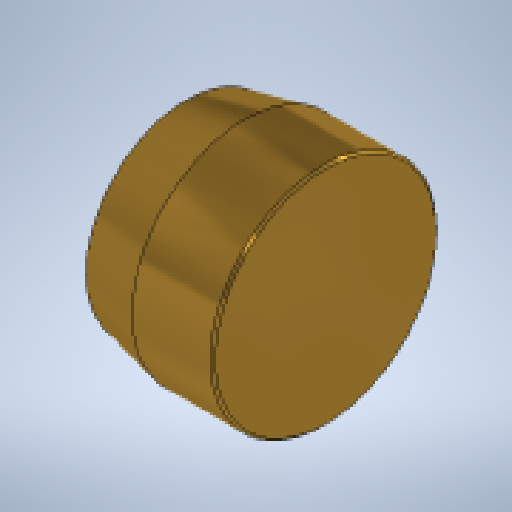
# Autodesk Inventor part: Flywheel
Saved by Autodesk Inventor 2023.2 (Build 272271000, 271)
## iProperties
Created: 2024-01-10
Part Number: Flywheel
Material: Brass, Soft Yellow
Document SubType Name: Modeling
Designer: Nathan Cai
Mass: 167.124 g
Surface Area: 93.7474 cm^2
Volume: 19.7313 cm^3
Density: 8.47 g/cm^3
Appearance: Brass - Satin
Author: Nathan Cai
Autodesk Inventor part; units mm, degrees
ref_plane "YZ Plane" through (0, 0, 0) normal (1, 0, 0) x (0, 1, 0)
ref_plane "XZ Plane" through (0, 0, 0) normal (0, 1, 0) x (-1, 0, 0)
ref_plane "XY Plane" through (0, 0, 0) normal (0, 0, 1) x (1, 0, 0)
sketch "Sketch1" plane through (0, 0, 0) normal (0, 1, 0) x (-1, 0, 0)
  line L0 (0, 0) -> (3.5, 0)
  line L1 (3.5, 0) -> (3.5, -8)
  line L2 (3.5, -8) -> (0, -8)
  line L3 (0, -8) -> (0, 0)
  line L4 (3.5, 0) -> (11.5, 0)
  line L5 (11.5, 0) -> (11.5, -13.9)
  line L6 (11.5, -13.9) -> (3.5, -13.9)
  line L7 (3.5, -13.9) -> (3.5, 0)
  line L8 (0, 0) -> (-13, 0)
  line L9 (-13, 0) -> (-13, -23)
  line L10 (-13, -23) -> (0, -23)
  line L11 (0, -23) -> (0, 0)
  line L12 (-13, -21) -> (0, -18.118)
  line L13 (-13, 0) -> (11.5, 0)
  line L14 (11.5, 0) -> (11.5, -23)
  line L15 (11.5, -23) -> (-13, -23)
  line L16 (-13, -23) -> (-13, 0)
  line L17 (-13, -23) -> (0, -20.118) construction
  line L18 (11.5, -23) -> (15.5, -23)
  line L19 (15.5, -23) -> (15.5, -18.5)
  line L20 (15.5, -18.5) -> (11.5, -18.5)
  line L21 (11.5, -18.5) -> (11.5, -23)
  line L22 (0, -8) -> (-5, -8)
  line L23 (-5, -8) -> (-5, -12)
  line L24 (-5, -12) -> (0, -12)
  line L25 (0, -12) -> (0, -8)
  line L26 (3.5, -8) -> (-2, -8)
  line L27 (-2, -8) -> (-2, -23)
  line L28 (-2, -23) -> (3.5, -23)
  line L29 (3.5, -23) -> (3.5, -8)
  line L30 (-5, -8) -> (-4, -8)
  line L31 (-4, -8) -> (-4, -9.1)
  line L32 (-4, -9.1) -> (-5, -9.1)
  line L33 (-5, -9.1) -> (-5, -8)
  line L34 (15.5, -20.3397) -> (3.5, -23)
  point P0 (3.5, -8)
  point P1 (0, -8)
  point P2 (0, -23)
  point P3 (11.5, -18.5)
  point P4 (0, -12)
  point P5 (0, -8)
  point P6 (0, -23)
  point P7 (3.5, -8)
  point P8 (-2, -12)
  point P9 (-2, -18.5614)
  point P10 (-4, -8)
  point P11 (-5, -9.1)
  point P12 (3.5, 0)
  point P13 (0, -12)
  dimension "d0" = 3.5
  dimension "d1" = 8
  dimension "d2" = 8
  dimension "d3" = 13.9
  dimension "d6" = 13
  dimension "d7" = 23
  dimension "d9" = 21
  dimension "d35" = 4
  dimension "d36" = 18.5
  dimension "d41" = 4
  dimension "d42" = 12.5
  dimension "d43" = 8.5
  dimension "d44" = 5.5
  dimension "d45" = 1
  dimension "d46" = 1.1
  constraints: 70 end point, 18 parallel, 8 horizontal, 8 perpendicular, 8 point on line
  measures "d0" distance of L1.end L2.end
  measures "d1" distance of L0.end L1.end
  measures "d2" distance of L5.end L6.end
  measures "d3" distance of L4.end L5.end
  measures "d6" distance of L10.end L9.end
  measures "d7" distance of L9.end L8.end
  measures "d9" distance from line of L8 L12.start
  measures "d35" distance of L20.end L19.end
  measures "d36" distance between parallel lines of L8 L20
  measures "d41" distance of L23.end L22.end
  measures "d42" angle of L15 L12
  measures "d43" distance between parallel lines of L7 L23
  measures "d44" distance between parallel lines of L29 L27
  measures "d45" distance of L31.end L32.end
  measures "d46" distance of L30.end L31.end
revolve "Revolution1" add sketch "Sketch1" angle 360 about axis through (0, 0, 0) along (-1, 0, 0) contours L2 L7 L29 L15 L11 | L11 L24 L27 L22 | L27 L24 L23 L32 L31 L22 | L12 L27 L10 L9 | L6 L14 L34 L29 | L11 L10 L27 L12 | L20 L19 L34 L14
chamfer "Chamfer2" distance 3.675 distance2 3.5875 1 edges at (-3.5, 0, 8) measured on face at (-3, 0, 8)
chamfer "Chamfer4" distance 0.5 angle 45 1 edges at (13, 0, 23)
chamfer "Chamfer5" distance 1.5 distance2 3 1 edges at (-11.5, 0, 13.9) measured on face at (-11, 0, 13.9)
sketch "Sketch5" plane through (13, 0, 0) normal (1, 0, 0) x (0, 0, -1)
  line L0 (-22, -22) -> (22, -22)
  line L1 (22, -22) -> (22, 22)
  line L2 (22, 22) -> (-22, 22)
  line L3 (-22, 22) -> (-22, -22)
  line L4 (-22, -22) -> (22, 22) construction
  line L5 (22, -22) -> (-22, 22) construction
  circle A0 centre (0, 0) radius 35
  point P0 (0, 0)
  dimension "d53" = 44
  dimension "d54" = 44
  dimension "d55" = 70
  constraints: 12 end point, 2 midpoint, 2 parallel, 1 centre point, 1 coincident, 1 horizontal, 1 perpendicular
  measures "d53" distance of L2.end L1.end
  measures "d54" distance of L1.end L0.end
  measures "d55" diameter of A0
equation "\"d53\" = d54"
body "Solid1"
